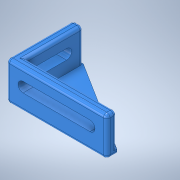
# Autodesk Inventor part: RightAngle_Bracket_60mm
Saved by Autodesk Inventor 2021 (Build 250183000, 183)
## iProperties
Created: 2021-02-10
Part Number: RightAngle_Bracket_60mm
Material: Generic
Document SubType Name: Modeling
Designer: Jorian Brusind
Density: 1 g/cm^3
Appearance: Cyan
Author: Jorian Brusind
Autodesk Inventor part; units mm, degrees
ref_plane "YZ Plane" through (0, 0, 0) normal (1, 0, 0) x (0, 1, 0)
ref_plane "XZ Plane" through (0, 0, 0) normal (0, 1, 0) x (-1, 0, 0)
ref_plane "XY Plane" through (0, 0, 0) normal (0, 0, 1) x (1, 0, 0)
sketch "Sketch1" plane through (0, 0, 0) normal (0, 1, 0) x (-1, 0, 0)
  line L0 (0, 0) -> (0, -40)
  line L1 (0, 0) -> (40, 0) construction
  line L2 (0, 0) -> (-60, 0)
  line L3 (-6, -40) -> (-6, -6)
  line L4 (-6, -6) -> (-60, -6)
  line L5 (-60, 0) -> (-60, -6)
  line L6 (0, -40) -> (-6, -40)
  line L7 (-60, -6) -> (-6, -40)
  dimension "d0" = 40
  dimension "d1" = 90
  dimension "d2" = 60
  dimension "d3" = 6
  constraints: 16 end point, 2 horizontal, 2 perpendicular, 2 vertical, 1 other
  measures "d0" distance of L0.start L0.end
  measures "d1" angle of L0 L1
  measures "d2" distance of L0.start L2.end
  measures "d3" distance between parallel lines of L0 L3
extrude "Extrusion1" add sketch "Sketch1" along normal blind 3
sketch "Sketch2" plane through (0, 3, 0) normal (0, 1, 0) x (1, 0, 0)
  line L0 (0, 40) -> (0, 0) projected
  line L1 (0, 0) -> (0, 40)
  line L2 (0, 0) -> (60, 0) projected
  line L3 (60, 0) -> (0, 0)
  line L4 (6, 40) -> (6, 0)
  line L5 (60, 6) -> (6, 6)
  line L6 (60, 6) -> (6, 40) projected
  line L7 (60, 6) -> (60, 0)
  line L8 (6, 40) -> (0, 40)
  dimension "d6" = 6
  constraints: 12 end point, 3 equal length, 3 perpendicular, 1 point on line
  measures "d6" distance between parallel lines of L0 L4
extrude "Extrusion2" add sketch "Sketch2" along normal blind 20 contours L8 L4 L2 L0 | L4 L5 L7 L2
sketch "Sketch3" plane through (6, 3, -6) normal (1, 0, 0) x (0, 0, -1)
  line L0 (34, 20) -> (-6, 20) projected
  line L1 (-6, 20) -> (4, 20)
  line L2 (4, 20) -> (4, 10)
  line L3 (4, 10) -> (24, 10) construction
  line L4 (4, 7) -> (24, 7)
  line L5 (24, 13) -> (4, 13)
  arc A0 (4, 13) -> (4, 7) centre (4, 10) ccw
  arc A1 (24, 7) -> (24, 13) centre (24, 10) ccw
  point P0 (-6, -3)
  point P1 (14, 10)
  dimension "d9" = 10
  dimension "d10" = 10
  dimension "d11" = 20
  dimension "d12" = 6
  constraints: 12 end point, 4 point on circle, 4 tangent, 2 centre point, 2 perpendicular, 1 midpoint, 1 parallel, 1 point on line
  measures "d9" distance of L0.end L1.end
  measures "d10" distance of L1.end L2.end
  measures "d11" distance of L2.end L3.end
  measures "d12" diameter of A1
extrude "Extrusion3" cut sketch "Sketch3" against normal blind 20
sketch "Sketch4" plane through (60, 3, -6) normal (0, 0, -1) x (-1, 0, 0)
  line L0 (10, 20) -> (10, 10)
  line L1 (10, 10) -> (50, 10) construction
  line L2 (10, 7) -> (50, 7)
  line L3 (50, 13) -> (10, 13)
  arc A0 (10, 13) -> (10, 7) centre (10, 10) ccw
  arc A1 (50, 7) -> (50, 13) centre (50, 10) ccw
  line L4 (60, -3) -> (60, 20) projected
  line L5 (0, 20) -> (54, 20) projected
  point P0 (30, 10)
  dimension "d16" = 10
  dimension "d17" = 40
  dimension "d18" = 6
  dimension "d35" = 10
  dimension "d36" = 13
  constraints: 10 end point, 4 point on circle, 4 tangent, 2 centre point, 1 horizontal, 1 midpoint, 1 parallel, 1 vertical
  measures "d16" distance of L0.start L0.end
  measures "d17" distance of L0.end L1.end
  measures "d18" diameter of A1
  measures "d35" distance from line of L4 L1.end
  measures "d36" distance between parallel lines of L5 L2
extrude "Extrusion4" cut sketch "Sketch4" against normal blind 20
fillet "Fillet1" radius 2 3 edges at (0, 11.5, 0) (60, 11.5, 0) (0, 11.5, -40)
fillet "Fillet2" radius 2 2 edges at (33, 23, -6) (6, 23, -23)
fillet "Fillet3" radius 2 11 edges at (59.4142, 23, -0.5858) (60, 23, -3) (60, 22.4142, -5.4142) (60, 12, -6) (0.5858, 23, -0.5858) (0, 23, -20) (0.5858, 23, -39.4142) (3, 23, -40) (5.4142, 22.4142, -40) (6, 12, -40) (30, 23, 0)
fillet "Fillet4" radius 2 7 edges at (0.5858, 0, -39.4142) (4, 0, -40) (0.5858, 0, -0.5858) (30, 0, 0) (59.4142, 0, -0.5858) (60, 0, -4) (0, 0, -20)
body "Solid1"
